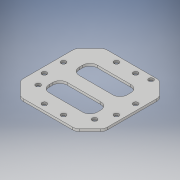
# Autodesk Inventor part: body_plate
Saved by Autodesk Inventor 2019 (Build 230136000, 136)
## iProperties
Created: 2019-01-09
Part Number: body_plate
Material: Generic
Document SubType Name: Modeling
Designer: Daniel
Density: 1 g/cm^3
Appearance: Default
Author: Daniel
Autodesk Inventor part; units mm, degrees
ref_plane "YZ Plane" through (0, 0, 0) normal (1, 0, 0) x (0, 1, 0)
ref_plane "XZ Plane" through (0, 0, 0) normal (0, 1, 0) x (-1, 0, 0)
ref_plane "XY Plane" through (0, 0, 0) normal (0, 0, 1) x (1, 0, 0)
sketch "Sketch23" plane through (0, 0, 0) normal (0, 1, 0) x (-1, 0, 0)
  line L0 (0, -49) -> (0, 49) projected
  line L1 (49, 0) -> (-49, 0) projected
  line L2 (35, -35) -> (-35, -35)
  line L3 (-35, -35) -> (-35, 35)
  line L4 (-35, 35) -> (35, 35)
  line L5 (35, 35) -> (35, -35)
  point P0 (0, 0)
  dimension "d310" = 70
  dimension "d311" = 70
  constraints: 8 end point, 2 parallel, 1 horizontal, 1 perpendicular, 2 other
  measures "d310" distance between parallel lines of L3 L5
  measures "d311" distance between parallel lines of L4 L2
extrude "Extrusion14" add sketch "Sketch23" along normal blind 2
sketch "Sketch37" plane through (0, 2, 0) normal (0, 1, 0) x (1, 0, 0)
  line L0 (-35, -35) -> (35, -35) projected
  line L1 (35, -35) -> (35, 35) projected
  line L2 (35, 35) -> (-35, 35) projected
  line L3 (-35, 35) -> (-35, -35) projected
  line L4 (-49, 0) -> (49, 0) projected
  line L5 (0, 49) -> (0, -49) projected
  line L6 (-26.65, 34.3) -> (26.65, 34.3) construction
  line L7 (26.65, 34.3) -> (26.65, -34.3) construction
  line L8 (26.65, -34.3) -> (-26.65, -34.3) construction
  line L9 (-26.65, -34.3) -> (-26.65, 34.3) construction
  point P0 (-24.15, -19)
  point P1 (24.15, -20.3)
  point P2 (19.05, 31.8)
  dimension "d327" = 68.6
  dimension "d328" = 53.3
  dimension "d329" = 15.3
  dimension "d330" = 14
  dimension "d331" = 2.5
  dimension "d332" = 2.5
  dimension "d333" = 2.5
  dimension "d334" = 7.6
  constraints: 8 end point, 2 parallel, 1 horizontal, 1 perpendicular, 2 other
  measures "d327" distance between parallel lines of L8 L6
  measures "d328" distance between parallel lines of L7 L9
  measures "d329" distance from line of L8 point (-24.15, -19)
  measures "d330" distance from line of L8 point (24.15, -20.3)
  measures "d331" distance from line of L7 point (24.15, -20.3)
  measures "d332" distance from line of L9 point (-24.15, -19)
  measures "d333" distance from line of L6 point (19.05, 31.8)
  measures "d334" distance from line of L7 point (19.05, 31.8)
hole "Hole18" at (-24.15, 2, 19) at (24.15, 2, 20.3) at (19.05, 2, -31.8) direction (0, -1, 0) diameter 4 end through all
sketch "Sketch40" plane through (0, 2, 0) normal (0, 1, 0) x (1, 0, 0)
  circle A0 centre (19.05, 31.8) radius 2 projected
  circle A1 centre (-24.15, -19) radius 2 projected
  circle A2 centre (24.15, -20.3) radius 2 projected
  line L0 (35, 35) -> (-35, 35) projected
  line L1 (-35, 35) -> (-35, -35) projected
  line L2 (-35, -35) -> (35, -35) projected
  line L3 (35, -35) -> (35, 35) projected
  line L4 (-49, 0) -> (49, 0) projected
  line L5 (0, 49) -> (0, -49) projected
  point P0 (0, 0)
  point P1 (8, 30)
  point P2 (30, 8)
  point P3 (30, -8)
  point P4 (-30, 8)
  point P5 (-30, -8)
  point P6 (-8, -30)
  point P7 (8, -30)
  point P8 (-8, 30)
  dimension "d445" = 8
  dimension "d446" = 5
  dimension "d447" = 8
  dimension "d448" = 5
  dimension "d449" = 8
  dimension "d450" = 5
  dimension "d458" = 8
  dimension "d459" = 8
  dimension "d460" = 5
  dimension "d461" = 5
  dimension "d462" = 5
  dimension "d463" = 8
  dimension "d464" = 8
  dimension "d465" = 5
  dimension "d478" = 8
  dimension "d479" = 5
  measures "d445" distance from line of L5 point (8, 30)
  measures "d446" distance from line of L0 point (8, 30)
  measures "d447" distance from line of L4 point (30, 8)
  measures "d448" distance from line of L3 point (30, 8)
  measures "d449" distance from line of L4 point (30, -8)
  measures "d450" distance from line of L3 point (30, -8)
  measures "d458" distance from line of L4 point (-30, 8)
  measures "d459" distance from line of L4 point (-30, -8)
  measures "d460" distance from line of L1 point (-30, -8)
  measures "d461" distance from line of L1 point (-30, 8)
  measures "d462" distance from line of L2 point (-8, -30)
  measures "d463" distance from line of L5 point (-8, -30)
  measures "d464" distance from line of L5 point (8, -30)
  measures "d465" distance from line of L2 point (8, -30)
  measures "d478" distance from line of L5 point (-8, 30)
  measures "d479" distance from line of L0 point (-8, 30)
sketch "Sketch41" plane through (0, 2, 0) normal (0, 1, 0) x (1, 0, 0)
  circle A0 centre (19.05, 31.8) radius 2 projected
  circle A1 centre (-24.15, -19) radius 2 projected
  circle A2 centre (24.15, -20.3) radius 2 projected
  line L0 (35, 35) -> (-35, 35) projected
  line L1 (-35, 35) -> (-35, -35) projected
  line L2 (-35, -35) -> (35, -35) projected
  line L3 (35, -35) -> (35, 35) projected
  line L4 (-49, 0) -> (49, 0) projected
  line L5 (0, 49) -> (0, -49) projected
  line L6 (-20, 20) -> (20, 20)
  line L7 (20, 20) -> (20, 5)
  line L8 (20, 5) -> (-20, 5)
  line L9 (-20, 5) -> (-20, 20)
  line L10 (-20, -5) -> (20, -5)
  line L11 (20, -5) -> (20, -20)
  line L12 (20, -20) -> (-20, -20)
  line L13 (-20, -20) -> (-20, -5)
  dimension "d467" = 10
  dimension "d468" = 40
  dimension "d480" = 15
  dimension "d481" = 15
  constraints: 16 end point, 4 parallel, 2 horizontal, 2 perpendicular, 1 collinear, 1 point on line, 2 other
  measures "d467" distance between parallel lines of L8 L10
  measures "d468" distance between parallel lines of L9 L7
  measures "d480" distance between parallel lines of L0 L6
  measures "d481" distance between parallel lines of L2 L12
hole "Hole21" at (8, 2, -30) at (30, 2, -8) at (30, 2, 8) at (-30, 2, -8) at (-30, 2, 8) at (-8, 2, 30) at (8, 2, 30) at (-8, 2, -30) direction (0, -1, 0) diameter 4 end through all
extrude "Extrusion25" cut sketch "Sketch41" against normal up to next contours L6 L7 L8 L5 | L5 L8 L9 L6 | L10 L11 L12 L5 | L5 L12 L13 L10
fillet "Fillet26" radius 6 8 edges at (20, 1, -20) (-20, 1, -20) (-20, 1, -5) (20, 1, -5) (20, 1, 5) (20, 1, 20) (-20, 1, 20) (-20, 1, 5)
chamfer "Chamfer10" distance 12 angle 45 4 edges at (-35, 1, 35) (35, 1, 35) (35, 1, -35) (-35, 1, -35)
fillet "Fillet27" radius 6 8 edges at (-23, 1, 35) (-35, 1, 23) (-35, 1, -23) (-23, 1, -35) (23, 1, -35) (35, 1, -23) (23, 1, 35) (35, 1, 23)
body "Solid5"
